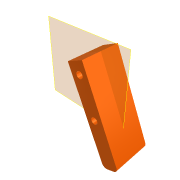
# Autodesk Inventor part: Gripper_linear_finger_long
Saved by Autodesk Inventor 2022 (Build 260153000, 153)
## iProperties
Created: 2023-01-05
Part Number: Gripper_linear_finger_long
Material: Generisch
Document SubType Name: Modeling
Designer: diederichbenedict
Density: 1 g/cm^3
Appearance: Glatt - Hellorange
Author: diederichbenedict
Autodesk Inventor part; units mm, degrees
ref_plane "YZ Plane" through (0, 0, 0) normal (1, 0, 0) x (0, 1, 0)
ref_plane "XZ Plane" through (0, 0, 0) normal (0, 1, 0) x (-1, 0, 0)
ref_plane "XY Plane" through (0, 0, 0) normal (0, 0, 1) x (1, 0, 0)
ref_plane "Arbeitsebene1" through (0, 0, 0) normal (0, 0, 1) x (1, 0, 0)
sketch "Skizze1" plane through (0, 0, 0) normal (0, 0, 1) x (1, 0, 0)
  line L0 (6, 5) -> (6, 20.6772) projected
  line L1 (25.0752, 5) -> (6, 5) projected
  line L2 (20.3151, 15.4507) -> (25.0752, 5)
  line L3 (6, 20.6772) -> (20.3151, 15.4507) projected
  circle A0 centre (28.7957, 2.7835) radius 1.4 projected
  circle A1 centre (22.3001, 17.2899) radius 1.4
  line L4 (32.7967, 0.1099) -> (23.0022, 21.6136)
  arc A2 (30.9766, -2.7191) -> (32.7967, 0.1099) centre (30.9766, -0.7191) ccw projected
  line L5 (29.8778, -2.7191) -> (30.9766, -2.7191) projected
  arc A3 (28.0577, -1.5481) -> (29.8778, -2.7191) centre (29.8778, -0.7191) ccw projected
  line L6 (27.3526, 0) -> (28.0577, -1.5481) projected
  line L7 (0, 0) -> (27.3526, 0) projected
  line L8 (0, 0) -> (0, 26) projected
  line L9 (0, 26) -> (6, 26) projected
  line L10 (23.0022, 21.6136) -> (18.452, 19.5411)
  line L11 (18.452, 19.5411) -> (34.0518, -14.708)
  line L12 (34.0518, -14.708) -> (38.602, -12.6355)
  line L13 (38.602, -12.6355) -> (23.0022, 21.6136)
  line L14 (23.4977, 22.9382) -> (17.1274, 20.0366)
  line L15 (17.1274, 20.0366) -> (32.7273, -14.2125)
  line L16 (35.3764, -15.2036) -> (38.1065, -13.96)
  line L17 (39.0976, -11.3109) -> (23.4977, 22.9382)
  arc A4 (38.1065, -13.96) -> (39.0976, -11.3109) centre (37.2775, -12.1399) ccw
  arc A5 (32.7273, -14.2125) -> (35.3764, -15.2036) centre (34.5474, -13.3835) ccw
  point P0 (22.6951, 10.2253)
  point P1 (28.0577, -1.5481)
  point P2 (26.2537, 0)
  point P3 (18.9971, 15.9319)
  dimension "d2" = 1
  dimension "d3" = 2
  constraints: 20 end point, 4 parallel, 4 point on circle, 4 tangent, 3 centre point, 2 perpendicular, 1 collinear, 1 equal radius, 1 midpoint, 1 point on line, 3 other
  measures "d2" distance between parallel lines of L13 L17
  measures "d3" radius of A4
extrude "Extrusion1" add sketch "Skizze1" along normal mid plane 16 contours L15 L3 L2 L1 | L1 L11 L7 L15 | L15 L14 L17 A4 L16 A5 L7 L6 L11 L12 L13 L4 L10 L3 | L2 L11 L10 L4 A2 L5 A3 L6 | A3 L5 A2 L13 L12 L11
